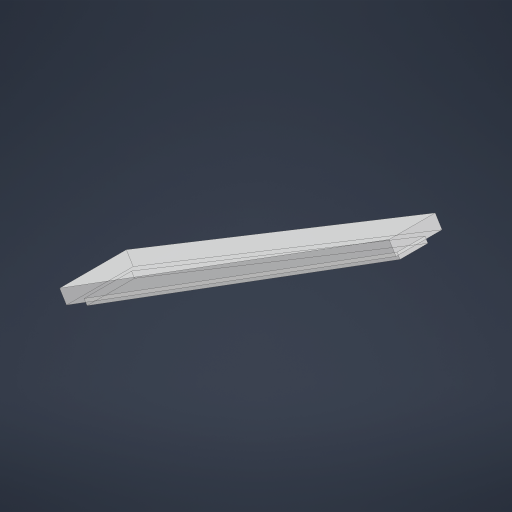
# Autodesk Inventor part: Touch Fifth
Saved by Autodesk Inventor 2023 (Build 270158000, 158)
## iProperties
Created: 2022-06-12
Part Number: Touch Fifth
Material: Polycarbonate, Smoke
Document SubType Name: Modeling
Designer: FizzyApple12
Density: 1.2 g/cm^3
Appearance: Polycarbonate - Semi Clear
Author: FizzyApple12
Autodesk Inventor part; units mm, degrees
ref_plane "XZ Plane" through (0, 0, 0) normal (0, 1, 0) x (-1, 0, 0)
ref_plane "XY Plane" through (0, 0, 0) normal (0, 0, 1) x (1, 0, 0)
sketch "Sketch1" plane through (0, 0, 0) normal (1, 0, 0) x (0, 1, 0)
  circle A0 centre (0, 0) radius 431.8 construction
  line L0 (-431.2082, -22.5987) -> (-431.2082, 22.5987)
  line L1 (-431.2082, -22.5987) -> (-386.0109, -22.5987) construction
  line L2 (-431.2082, -22.5987) -> (0, 0) construction
  line L3 (0, 0) -> (-431.2082, 22.5987) construction
  dimension "d0" = 863.6
  dimension "d3" = 90
  dimension "d4" = 6
  constraints: 8 end point, 2 point on circle, 1 centre point, 1 coincident, 1 horizontal, 1 perpendicular
  measures "d0" diameter of A0
  measures "d3" angle of L1 L0
  measures "d4" angle of L3 L2
ref_plane "Work Plane1" through (216.1794, 0, 0) normal (1, 0, 0) x (0, 1, 0)
sketch "Sketch2" plane through (216.1794, 0, 0) normal (1, 0, 0) x (0, 1, 0)
  circle A0 centre (0, 0) radius 298.45 construction
  line L0 (-298.041, 15.6197) -> (-298.041, -15.6197)
  line L1 (-298.041, 15.6197) -> (-266.8017, 15.6197) construction
  line L2 (-298.041, 15.6197) -> (0, 0) construction
  line L3 (0, 0) -> (-298.041, -15.6197) construction
  dimension "d2" = 596.9
  dimension "d5" = 90
  dimension "d6" = 6
  constraints: 8 end point, 2 point on circle, 1 centre point, 1 coincident, 1 horizontal, 1 perpendicular
  measures "d2" diameter of A0
  measures "d5" angle of L0 L1
  measures "d6" angle of L3 L2
ref_plane "Work Plane2" through (0, -431.2082, -22.5987) normal (-0.5244795, 0.8514231, 0) x (0, 0, 1)
sketch "Sketch3" plane through (0, -431.2082, -22.5987) normal (-0.5244795, 0.8514231, 0) x (0, 0, 1)
  line L0 (0, 0) -> (45.1973, 0) projected
  line L1 (38.2183, 253.9036) -> (6.979, 253.9036) projected
  line L2 (6.979, 253.9036) -> (0, 0)
  line L3 (45.1973, 0) -> (38.2183, 253.9036)
  point P0 (22.5987, 226.1599)
  constraints: 4 end point
extrude "Extrusion1" add sketch "Sketch3" against normal blind 12.7
sketch "Sketch4" plane through (6.6609, -442.0213, -22.5987) normal (0.5244795, -0.8514231, 0) x (0.8514231, 0.5244795, 0)
  line L0 (6.35, 6.5269) -> (6.35, 38.6704)
  line L1 (6.35, 38.6704) -> (247.5536, 32.0405)
  line L2 (247.5536, 32.0405) -> (247.5536, 13.1569)
  line L3 (247.5536, 13.1569) -> (6.35, 6.5269)
  line L4 (0, 45.1973) -> (0, 0) projected
  line L5 (253.9036, 38.2183) -> (0, 45.1973) projected
  line L6 (0, 0) -> (253.9036, 6.979) projected
  line L7 (253.9036, 6.979) -> (253.9036, 38.2183) projected
  point P0 (226.1599, 22.5987)
  dimension "d9" = 6.35
  dimension "d10" = 6.35
  dimension "d11" = 6.35
  dimension "d12" = 6.35
  constraints: 8 end point, 4 parallel
  measures "d9" distance between parallel lines of L4 L0
  measures "d10" distance between parallel lines of L6 L3
  measures "d11" distance between parallel lines of L5 L1
  measures "d12" distance between parallel lines of L7 L2
extrude "Extrusion2" cut sketch "Sketch4" against normal blind 3.81
body "Solid1"
